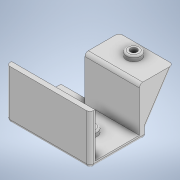
# Autodesk Inventor part: cornerMountR_PBF
Saved by Autodesk Inventor 2020 (Build 240168000, 168)
## iProperties
Created: 2020-01-08
Part Number: cornerMountR_PBF
Material: Generic
Document SubType Name: Modeling
Designer: PAB
Density: 1 g/cm^3
Appearance: Default
Author: PAB
Autodesk Inventor part; units mm, degrees
ref_plane "YZ Plane" through (0, 0, 0) normal (1, 0, 0) x (0, 1, 0)
ref_plane "XZ Plane" through (0, 0, 0) normal (0, 1, 0) x (-1, 0, 0)
ref_plane "XY Plane" through (0, 0, 0) normal (0, 0, 1) x (1, 0, 0)
sketch "Sketch1" plane through (0, 0, 0) normal (0, 1, 0) x (-1, 0, 0)
  line L0 (20.5, 16.2) -> (-20.5, 16.2)
  line L1 (-20.5, 16.2) -> (-20.5, -16.2)
  line L2 (-20.5, -16.2) -> (20.5, -16.2)
  line L3 (20.5, -16.2) -> (20.5, 16.2)
  point P0 (0, 0)
  dimension "d0" = 41
  dimension "d1" = 32.4
  constraints: 8 end point, 2 parallel, 1 horizontal, 1 perpendicular
  measures "d0" distance of L2.end L1.end
  measures "d1" distance of L1.end L0.end
extrude "Extrusion1" add sketch "Sketch1" along normal blind 3
sketch "Sketch4" plane through (20.5, 0, -16.2) normal (0, 0, -1) x (-1, 0, 0)
  line L0 (41, 3) -> (0, 3) projected
  line L1 (0, 28.4) -> (41, 28.4) projected
  line L2 (0, 3) -> (21.5, 3)
  line L3 (21.5, 3) -> (21.5, 28.4)
  line L4 (21.5, 28.4) -> (0, 28.4)
  line L5 (0, 28.4) -> (0, 3)
  point P0 (20.5, 0)
  dimension "d12" = 21.5
  constraints: 8 end point, 2 parallel, 1 horizontal, 1 perpendicular, 1 point on line
  measures "d12" distance of L4.end L3.end
extrude "Extrusion4" cut sketch "Sketch4" against normal blind 3
sketch "Sketch5" plane through (-20.5, 0, 16.2) normal (0, 0, 1) x (1, 0, 0)
  line L0 (41, 28.4) -> (0, 28.4) projected
  line L1 (41, 3) -> (0, 3) projected
  line L2 (0, 28.4) -> (21.5, 28.4)
  line L3 (21.5, 28.4) -> (21.5, 3)
  line L4 (21.5, 3) -> (0, 3)
  line L5 (0, 3) -> (0, 28.4)
  point P0 (20.5, 0)
  point P1 (19.5, 3)
  point P2 (19.5, 3)
  dimension "d15" = 21.5
  constraints: 8 end point, 2 parallel, 1 horizontal, 1 perpendicular, 1 point on line
  measures "d15" distance of L3.end L1.end
extrude "Extrusion5" cut sketch "Sketch5" against normal blind 3
sketch "Sketch6" plane through (0, 3, 0) normal (0, 1, 0) x (1, 0, 0)
  circle A0 centre (13, 0) radius 4.25
  circle A1 centre (-13, 0) radius 4.25
  point P0 (0, 0)
  dimension "d20" = 8.5
  dimension "d21" = 8.5
  constraints: 2 centre point
  measures "d20" diameter of A0
  measures "d21" diameter of A1
extrude "Extrusion6" add sketch "Sketch6" along normal blind 3
sketch "Sketch7" plane through (0, 0, 0) normal (0, -1, 0) x (1, 0, 0)
  circle A0 centre (-13, 0) radius 4.25 projected
  circle A1 centre (-13, 0) radius 2
  circle A2 centre (13, 0) radius 4.25 projected
  circle A3 centre (13, 0) radius 2
  point P0 (0, 0)
  dimension "d24" = 4
  dimension "d25" = 4
  constraints: 2 centre point, 2 coincident
  measures "d24" diameter of A1
  measures "d25" diameter of A3
extrude "Extrusion7" cut sketch "Sketch7" against normal blind 6 contours A1 | A3
sketch "Sketch8" plane through (0, 0, 0) normal (0, -1, 0) x (1, 0, 0)
  circle A0 centre (-13, 0) radius 2 projected
  circle A1 centre (-13, 0) radius 3
  circle A2 centre (13, 0) radius 2 projected
  circle A3 centre (13, 0) radius 3
  point P0 (0, 0)
  dimension "d28" = 6
  dimension "d29" = 6
  constraints: 2 centre point, 2 coincident
  measures "d28" diameter of A1
  measures "d29" diameter of A3
extrude "Extrusion8" cut sketch "Sketch8" against normal blind 3 contours A0 | A1 | A2 | A3
sketch "Sketch15" plane through (20.5, 0, 16.2) normal (1, 0, 0) x (0, 0, -1)
  line L0 (0, 3) -> (32.4, 3) projected
  line L1 (0, 0) -> (32.4, 0)
  line L2 (32.4, 0) -> (32.4, 3)
  line L3 (32.4, 3) -> (0, 3)
  line L4 (0, 3) -> (0, 0)
  point P0 (16.2, 0)
  constraints: 8 end point, 2 parallel, 1 horizontal, 1 perpendicular
extrude "Extrusion15" add sketch "Sketch15" along normal blind 8.7
sketch "Sketch23" plane through (0, 3, 0) normal (0, 1, 0) x (1, 0, 0)
  line L0 (-20.5, 16.2) -> (29.2, 16.2) projected
  line L1 (29.2, 16.2) -> (-3.2, 16.2)
  line L2 (-3.2, 16.2) -> (-3.2, 13.2)
  line L3 (-3.2, 13.2) -> (29.2, 13.2)
  line L4 (29.2, 13.2) -> (29.2, 16.2)
  point P0 (0, 0)
  dimension "d81" = 32.4
  dimension "d82" = 3
  constraints: 8 end point, 2 parallel, 1 horizontal, 1 perpendicular
  measures "d81" distance of L3.end L2.end
  measures "d82" distance of L2.end L1.end
extrude "Extrusion23" add sketch "Sketch23" along normal blind 26.4
sketch "Sketch24" plane through (-20.5, 0, -16.2) normal (0, 0, -1) x (-1, 0, 0)
  line L0 (-17.3, 3) -> (-17.3, 29.4) projected
  line L1 (-49.7, 3) -> (-17.3, 3) projected
  line L2 (-17.3, 29.4) -> (-20.3, 29.4)
  line L3 (-20.3, 29.4) -> (-20.3, 3)
  line L4 (-20.3, 3) -> (-17.3, 3)
  line L5 (-17.3, 3) -> (-17.3, 29.4)
  line L6 (-49.7, 0) -> (-49.7, 29.4) projected
  line L7 (-49.7, 29.4) -> (-46.7, 29.4)
  line L8 (-46.7, 29.4) -> (-46.7, 3)
  line L9 (-46.7, 3) -> (-49.7, 3)
  line L10 (-49.7, 3) -> (-49.7, 29.4)
  line L11 (-20.3, 29.4) -> (-46.7, 29.4)
  line L12 (-46.7, 29.4) -> (-46.7, 26.4)
  line L13 (-46.7, 26.4) -> (-20.3, 26.4)
  line L14 (-20.3, 26.4) -> (-20.3, 29.4)
  point P0 (-20.5, 0)
  dimension "d85" = 3
  dimension "d86" = 3
  dimension "d87" = 3
  constraints: 24 end point, 6 parallel, 3 horizontal, 3 perpendicular, 3 point on line
  measures "d85" distance of L4.end L3.end
  measures "d86" distance of L8.end L9.end
  measures "d87" distance of L12.end L11.end
extrude "Extrusion24" add sketch "Sketch24" along normal blind 17.3 contours L1 L3 L2 L0 | L3 L13 L8 L11 | L1 L6 L7 L8
sketch "Sketch25" plane through (-3.2, 3, -13.2) normal (-1, 0, 0) x (0, 0, 1)
  line L0 (0, 26.4) -> (-20.3, 26.4) projected
  line L1 (0, 0) -> (-3, 0) projected
  line L2 (-20.3, 26.4) -> (-3, 0)
  line L3 (-20.3, 26.4) -> (-20.3, 0) projected
  line L4 (-3, 0) -> (-20.3, 0)
  line L5 (-20.3, 0) -> (-20.3, 26.4)
  point P0 (13.2, -3)
  constraints: 6 end point, 1 collinear, 1 perpendicular
extrude "Extrusion25" cut sketch "Sketch25" against normal blind 32.4
sketch "Sketch26" plane through (0, 29.4, 0) normal (0, 1, 0) x (1, 0, 0)
  circle A0 centre (13, 26) radius 2
  point P0 (0, 0)
  dimension "d92" = 4
  constraints: 1 centre point
  measures "d92" diameter of A0
extrude "Extrusion26" cut sketch "Sketch26" against normal blind 32.4
sketch "Sketch27" plane through (0, 29.4, 0) normal (0, 1, 0) x (1, 0, 0)
  circle A0 centre (13, 26) radius 2 projected
  circle A1 centre (13, 26) radius 4.25
  point P0 (0, 0)
  dimension "d95" = 8.5
  constraints: 1 centre point, 1 coincident
  measures "d95" diameter of A1
extrude "Extrusion27" add sketch "Sketch27" along normal blind 3
sketch "Sketch28" plane through (0, 3, 0) normal (0, 1, 0) x (1, 0, 0)
  line L0 (-20.5, -16.2) -> (29.2, -16.2) projected
  line L1 (-20.5, 16.2) -> (-20.5, -16.2) projected
  line L2 (29.2, -16.2) -> (-20.5, -16.2)
  line L3 (-20.5, -16.2) -> (-20.5, -13.2)
  line L4 (-20.5, -13.2) -> (29.2, -13.2)
  line L5 (29.2, -13.2) -> (29.2, -16.2)
  point P0 (0, 0)
  dimension "d98" = 3
  constraints: 8 end point, 2 parallel, 1 horizontal, 1 perpendicular, 1 point on line
  measures "d98" distance of L2.end L3.end
extrude "Extrusion28" add sketch "Sketch28" along normal blind 26.4
fillet "Fillet3" radius 1 3 edges at (8.75, 32.4, -26) (-17.25, 6, 0) (8.75, 6, 0)
fillet "Fillet4" radius 2 9 edges at (4.35, 0, 16.2) (-20.5, 0, 0) (29.2, 14.7, 16.2) (29.2, 0, 0) (29.2, 16.2, -24.85) (-3.2, 16.2, -24.85) (4.35, 0, -16.2) (13, 26.4, -31.5341) (-20.5, 14.7, 16.2)
sketch "Sketch29" plane through (-0.2, 26.4, -16.2) normal (0, -1, 0) x (1, 0, 0)
  circle A0 centre (13.2, -9.8) radius 2 projected
  circle A1 centre (13.2, -9.8) radius 3
  point P0 (0.2, 16.2)
  dimension "d103" = 6
  constraints: 1 centre point, 1 coincident
  measures "d103" diameter of A1
extrude "Extrusion29" cut sketch "Sketch29" against normal blind 3
fillet "Fillet5" radius 2 1 edges at (13, 29.4, -13.2)
body "Solid1"
